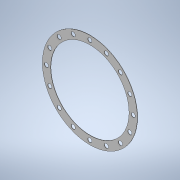
# Autodesk Inventor part: Прокладка крышек цилиндра
Saved by Autodesk Inventor 2021 (Build 250183000, 183)
## iProperties
Created: 2020-11-14
Part Number: Прокладка крышек цилиндра
Material: Типовые
Document SubType Name: Modeling
Designer: Тимоха
Density: 1 g/cm^3
Appearance: По умолчанию
Author: Тимоха
Autodesk Inventor part; units mm, degrees
ref_plane "YZ Plane" through (0, 0, 0) normal (1, 0, 0) x (0, 1, 0)
ref_plane "XZ Plane" through (0, 0, 0) normal (0, 1, 0) x (-1, 0, 0)
ref_plane "XY Plane" through (0, 0, 0) normal (0, 0, 1) x (1, 0, 0)
sketch "Эскиз1" plane through (0, 0, 0) normal (0, 0, 1) x (1, 0, 0)
  circle A0 centre (0, 0) radius 240
  circle A1 centre (0, 0) radius 290
  dimension "d0" = 480
  dimension "d1" = 580
  constraints: 2 centre point, 2 coincident
  measures "d0" diameter of A0
  measures "d1" diameter of A1
extrude "Выдавливание1" add sketch "Эскиз1" along normal blind 2
sketch "Эскиз2" plane through (0, 0, 2) normal (0, 0, 1) x (1, 0, 0)
  circle A0 centre (0, 0) radius 290 projected
  line L0 (0, 290) -> (0, 265)
  dimension "d4" = 25
  constraints: 2 end point, 1 vertical, 1 vertical alignment, 1 other
  measures "d4" distance of L0.start L0.end
hole "Отверстие1" at (0, 265, 2) direction (0, 0, -1) diameter 26 end through all
pattern_circular "Круговой массив1" count 16 over 360 about axis through (0, 0, -10) along (0, 0, 1) of "Отверстие1"
